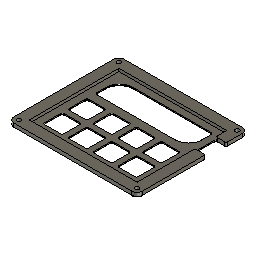
combined (Autodesk Fusion 360 archive; units mm, degrees)
design "Case_Lid"
Autodesk Fusion 360 part; units mm, degrees
sketch "plate-2025-12-06T19_36_10.325Z" plane through (0, 0, 0) normal (0, 0, 1) x (1, 0, 0)
  line L0 (3.275, -2.525) -> (15.775, -2.525)
  line L1 (3.275, -16.525) -> (15.775, -16.525)
  line L2 (2.525, -3.275) -> (2.525, -15.775)
  line L3 (16.525, -3.275) -> (16.525, -15.775)
  arc A0 (3.275, -2.525) -> (2.525, -3.275) centre (3.275, -3.275) ccw
  arc A1 (16.525, -3.275) -> (15.775, -2.525) centre (15.775, -3.275) ccw
  arc A2 (2.525, -15.775) -> (3.275, -16.525) centre (3.275, -15.775) ccw
  arc A3 (15.775, -16.525) -> (16.525, -15.775) centre (15.775, -15.775) ccw
  line L4 (22.325, -2.525) -> (34.825, -2.525)
  line L5 (22.325, -16.525) -> (34.825, -16.525)
  line L6 (21.575, -3.275) -> (21.575, -15.775)
  line L7 (35.575, -3.275) -> (35.575, -15.775)
  arc A4 (22.325, -2.525) -> (21.575, -3.275) centre (22.325, -3.275) ccw
  arc A5 (35.575, -3.275) -> (34.825, -2.525) centre (34.825, -3.275) ccw
  arc A6 (21.575, -15.775) -> (22.325, -16.525) centre (22.325, -15.775) ccw
  arc A7 (34.825, -16.525) -> (35.575, -15.775) centre (34.825, -15.775) ccw
  line L8 (41.375, -2.525) -> (53.875, -2.525)
  line L9 (41.375, -16.525) -> (53.875, -16.525)
  line L10 (40.625, -3.275) -> (40.625, -15.775)
  line L11 (54.625, -3.275) -> (54.625, -15.775)
  arc A8 (41.375, -2.525) -> (40.625, -3.275) centre (41.375, -3.275) ccw
  arc A9 (54.625, -3.275) -> (53.875, -2.525) centre (53.875, -3.275) ccw
  arc A10 (40.625, -15.775) -> (41.375, -16.525) centre (41.375, -15.775) ccw
  arc A11 (53.875, -16.525) -> (54.625, -15.775) centre (53.875, -15.775) ccw
  line L12 (60.425, -2.525) -> (72.925, -2.525)
  line L13 (60.425, -16.525) -> (72.925, -16.525)
  line L14 (59.675, -3.275) -> (59.675, -15.775)
  line L15 (73.675, -3.275) -> (73.675, -15.775)
  arc A12 (60.425, -2.525) -> (59.675, -3.275) centre (60.425, -3.275) ccw
  arc A13 (73.675, -3.275) -> (72.925, -2.525) centre (72.925, -3.275) ccw
  arc A14 (59.675, -15.775) -> (60.425, -16.525) centre (60.425, -15.775) ccw
  arc A15 (72.925, -16.525) -> (73.675, -15.775) centre (72.925, -15.775) ccw
  line L16 (3.275, -21.575) -> (15.775, -21.575)
  line L17 (3.275, -35.575) -> (15.775, -35.575)
  line L18 (2.525, -22.325) -> (2.525, -34.825)
  line L19 (16.525, -22.325) -> (16.525, -34.825)
  arc A16 (3.275, -21.575) -> (2.525, -22.325) centre (3.275, -22.325) ccw
  arc A17 (16.525, -22.325) -> (15.775, -21.575) centre (15.775, -22.325) ccw
  arc A18 (2.525, -34.825) -> (3.275, -35.575) centre (3.275, -34.825) ccw
  arc A19 (15.775, -35.575) -> (16.525, -34.825) centre (15.775, -34.825) ccw
  line L20 (22.325, -21.575) -> (34.825, -21.575)
  line L21 (22.325, -35.575) -> (34.825, -35.575)
  line L22 (21.575, -22.325) -> (21.575, -34.825)
  line L23 (35.575, -22.325) -> (35.575, -34.825)
  arc A20 (22.325, -21.575) -> (21.575, -22.325) centre (22.325, -22.325) ccw
  arc A21 (35.575, -22.325) -> (34.825, -21.575) centre (34.825, -22.325) ccw
  arc A22 (21.575, -34.825) -> (22.325, -35.575) centre (22.325, -34.825) ccw
  arc A23 (34.825, -35.575) -> (35.575, -34.825) centre (34.825, -34.825) ccw
  line L24 (41.375, -21.575) -> (53.875, -21.575)
  line L25 (41.375, -35.575) -> (53.875, -35.575)
  line L26 (40.625, -22.325) -> (40.625, -34.825)
  line L27 (54.625, -22.325) -> (54.625, -34.825)
  arc A24 (41.375, -21.575) -> (40.625, -22.325) centre (41.375, -22.325) ccw
  arc A25 (54.625, -22.325) -> (53.875, -21.575) centre (53.875, -22.325) ccw
  arc A26 (40.625, -34.825) -> (41.375, -35.575) centre (41.375, -34.825) ccw
  arc A27 (53.875, -35.575) -> (54.625, -34.825) centre (53.875, -34.825) ccw
  line L28 (60.425, -21.575) -> (72.925, -21.575)
  line L29 (60.425, -35.575) -> (72.925, -35.575)
  line L30 (59.675, -22.325) -> (59.675, -34.825)
  line L31 (73.675, -22.325) -> (73.675, -34.825)
  arc A28 (60.425, -21.575) -> (59.675, -22.325) centre (60.425, -22.325) ccw
  arc A29 (73.675, -22.325) -> (72.925, -21.575) centre (72.925, -22.325) ccw
  arc A30 (59.675, -34.825) -> (60.425, -35.575) centre (60.425, -34.825) ccw
  arc A31 (72.925, -35.575) -> (73.675, -34.825) centre (72.925, -34.825) ccw
  line L32 (-11.361, 35.925) -> (87.639, 35.925)
  line L33 (87.639, 35.925) -> (87.639, -49.075)
  line L34 (87.639, -49.075) -> (-11.361, -49.075)
  line L35 (-11.361, -49.075) -> (-11.361, 35.925)
  circle A32 centre (-7.361, 31.925) radius 1.6
  circle A33 centre (83.639, 31.925) radius 1.6
  circle A34 centre (83.639, -45.075) radius 1.6
  circle A35 centre (-7.361, -45.075) radius 1.6
  line L36 (73.753, 22.425) -> (12.525, 22.425)
  line L37 (2.525, 12.425) -> (2.525, 4.425)
  line L38 (2.525, 4.425) -> (63.753, 4.425)
  line L39 (73.753, 14.425) -> (73.753, 22.425)
  arc A36 (12.525, 22.425) -> (2.525, 12.425) centre (12.525, 12.425) ccw
  arc A37 (63.753, 4.425) -> (73.753, 14.425) centre (63.753, 14.425) ccw
  line L40 (-3.361, 27.925) -> (79.639, 27.925)
  line L41 (79.639, 27.925) -> (79.639, -41.075)
  line L42 (79.639, -41.075) -> (-3.361, -41.075)
  line L43 (-3.361, -41.075) -> (-3.361, 27.925)
  dimension "d1" = 99
  dimension "d2" = 85
  dimension "d3" = 13.886
  dimension "d4" = 13.5
  dimension "d12" = 3.2
  dimension "d13" = 4
  dimension "d14" = 4
  dimension "d15" = 3.2
  dimension "d16" = 4
  dimension "d17" = 4
  dimension "d18" = 3.2
  dimension "d19" = 3.2
  dimension "d20" = 4
  dimension "d21" = 4
  dimension "d22" = 4
  dimension "d23" = 4
  dimension "d34" = 13.886
  dimension "d36" = 13.886
  dimension "d37" = 18
  dimension "d38" = 13.5
  dimension "d39" = 10
  dimension "d40" = 10
  dimension "d47" = 8
  dimension "d48" = 8
  dimension "d49" = 8
  dimension "d50" = 8
  constraint horizontal L32
  constraint vertical L33
  constraint horizontal L34
  constraint vertical L35
  constraint horizontal L36
  constraint vertical L37
  constraint horizontal L38
  constraint vertical L39
  constraint tangent L36 A36
  constraint tangent L37 A36
  constraint tangent L38 A37
  constraint tangent L39 A37
  constraint horizontal L40
  constraint vertical L41
  constraint horizontal L42
  constraint vertical L43
  measures "d1" distance of L32.start L32.end
  measures "d2" distance of L32.start L34.end
  measures "d3" distance of L18 L35
  measures "d4" distance of L17 L34
  measures "d12" diameter of A32
  measures "d13" distance of L32 A32.centre
  measures "d14" distance of L35 A32.centre
  measures "d15" diameter of A33
  measures "d16" distance of L33 A33.centre
  measures "d17" distance of L32 A33.centre
  measures "d18" diameter of A35
  measures "d19" diameter of A34
  measures "d20" distance of L34 A34.centre
  measures "d21" distance of L33 A34.centre
  measures "d22" distance of L34 A35.centre
  measures "d23" distance of L35 A35.centre
  measures "d34" distance of L35 L37
  measures "d36" distance of L33 L39
  measures "d37" distance of L36 L38
  measures "d38" distance of L32 L36
  measures "d39" radius of A36
  measures "d40" radius of A37
  measures "d47" distance of L32 L40
  measures "d48" distance of L35 L43
  measures "d49" distance of L33 L41
  measures "d50" distance of L34 L42
extrude "Extrude1" add sketch "plate-2025-12-06T19_36_10.325Z" along normal blind 1.5 contours L32 L33 L34 L35 | L40 L41 L42 L43
extrude "Extrude2" add sketch "plate-2025-12-06T19_36_10.325Z" along normal blind 3.75 contours L32 L33 L34 L35
sketch "Sketch2" plane through (0, 0, 3.75) normal (0, 0, 1) x (-1, 0, 0)
  circle A0 centre (-83.639, -31.925) radius 1.6
  circle A1 centre (7.361, 45.075) radius 1.6
  line L0 (-79.639, 41.075) -> (3.361, 41.075)
  line L1 (3.361, 41.075) -> (3.361, -27.925)
  line L2 (3.361, -27.925) -> (-79.639, -27.925)
  line L3 (-79.639, -27.925) -> (-79.639, 41.075)
  circle A2 centre (-83.639, 45.075) radius 1.6
  circle A3 centre (7.361, -31.925) radius 1.6
  line L4 (11.361, 49.075) -> (-87.639, 49.075)
  line L5 (-87.639, 49.075) -> (-87.639, -35.925)
  line L6 (-87.639, -35.925) -> (11.361, -35.925)
  line L7 (11.361, -35.925) -> (11.361, 49.075)
  line L8 (-79.639, -19.549) -> (-87.639, -19.549)
  line L9 (-87.639, -19.549) -> (-87.639, -3.549)
  line L10 (-87.639, -3.549) -> (-79.639, -3.549)
  line L11 (-79.639, -3.549) -> (-79.639, -19.549)
  dimension "d67" = 16.376
  dimension "d68" = 52.624
  constraint horizontal L8
  constraint vertical L9
  constraint horizontal L10
  constraint vertical L11
  constraint coincident L5 L9.end
  constraint coincident L3 L8.start
  measures "d67" distance of L6 L8
  measures "d68" distance of L4 L10
extrude "Extrude4" cut sketch "Sketch2" against normal blind 5 contours L3 L5 L8 L9 L10 L11
fillet "Fillet11" radius 1 4 edges at (73.753, 22.425, 0.75) (2.525, 4.425, 0.75) (79.639, 3.549, 0.75) (79.639, 19.549, 0.75)
fillet "Fillet8" radius 4 4 edges at (87.639, 35.925, 1.875) (87.639, -49.075, 1.875) (-11.361, 35.925, 1.875) (-11.361, -49.075, 1.875)
fillet "Fillet9" radius 1 90 edges at (2.525, 8.925, 0) (5.4539, 19.4961, 0) (42.639, 22.425, 0) (73.4601, 22.1321, 0) (73.753, 17.925, 0) (70.8241, 7.3539, 0) (33.639, 4.425, 0) (2.8179, 4.7179, 0) (16.525, -9.525, 0) (16.3053, -16.3053, 0) (9.525, -16.525, 0) (2.7447, -16.3053, 0) (2.525, -9.525, 0) (2.7447, -2.7447, 0) (9.525, -2.525, 0) (16.3053, -2.7447, 0) (35.575, -9.525, 0) (35.3553, -16.3053, 0) (28.575, -16.525, 0) (21.7947, -16.3053, 0) (21.575, -9.525, 0) (21.7947, -2.7447, 0) (28.575, -2.525, 0) (35.3553, -2.7447, 0) (54.625, -9.525, 0) (54.4053, -16.3053, 0) (47.625, -16.525, 0) (40.8447, -16.3053, 0) (40.625, -9.525, 0) (40.8447, -2.7447, 0) (47.625, -2.525, 0) (54.4053, -2.7447, 0) (73.675, -9.525, 0) (73.4553, -16.3053, 0) (66.675, -16.525, 0) (59.8947, -16.3053, 0) (59.675, -9.525, 0) (59.8947, -2.7447, 0) (66.675, -2.525, 0) (73.4553, -2.7447, 0) (59.675, -28.575, 0) (59.8947, -21.7947, 0) (66.675, -21.575, 0) (73.4553, -21.7947, 0) (73.675, -28.575, 0) (73.4553, -35.3553, 0) (66.675, -35.575, 0) (59.8947, -35.3553, 0) (40.625, -28.575, 0) (40.8447, -21.7947, 0) (47.625, -21.575, 0) (54.4053, -21.7947, 0) (54.625, -28.575, 0) (54.4053, -35.3553, 0) (47.625, -35.575, 0) (40.8447, -35.3553, 0) (21.575, -28.575, 0) (21.7947, -21.7947, 0) (28.575, -21.575, 0) (35.3553, -21.7947, 0) (35.575, -28.575, 0) (35.3553, -35.3553, 0) (28.575, -35.575, 0) (21.7947, -35.3553, 0) (2.525, -28.575, 0) (2.7447, -21.7947, 0) (9.525, -21.575, 0) (16.3053, -21.7947, 0) (16.525, -28.575, 0) (16.3053, -35.3553, 0) (9.525, -35.575, 0) (2.7447, -35.3553, 0) (86.4674, 34.7534, 0) (38.139, 35.925, 0) (-10.1894, 34.7534, 0) (-11.361, -6.575, 0) (-10.1894, -47.9034, 0) (38.139, -49.075, 0) (86.4674, -47.9034, 0) (87.639, -20.763, 0) (87.639, 25.737, 0) (84.139, 19.549, 0) (79.9319, 19.2561, 0) (79.639, 11.549, 0) (79.9319, 3.8419, 0) (84.139, 3.549, 0) (87.639, 3.549, 1.875) (87.639, 19.549, 1.875) (79.639, 3.549, 2.625) (79.639, 19.549, 2.625)
fillet "Fillet12" radius 0.4 75 edges at (59.675, -28.575, 1.5) (59.8947, -21.7947, 1.5) (66.675, -21.575, 1.5) (73.4553, -21.7947, 1.5) (73.675, -28.575, 1.5) (73.4553, -35.3553, 1.5) (66.675, -35.575, 1.5) (59.8947, -35.3553, 1.5) (40.625, -28.575, 1.5) (40.8447, -21.7947, 1.5) (47.625, -21.575, 1.5) (54.4053, -21.7947, 1.5) (54.625, -28.575, 1.5) (54.4053, -35.3553, 1.5) (47.625, -35.575, 1.5) (40.8447, -35.3553, 1.5) (21.575, -28.575, 1.5) (21.7947, -21.7947, 1.5) (28.575, -21.575, 1.5) (35.3553, -21.7947, 1.5) (35.575, -28.575, 1.5) (35.3553, -35.3553, 1.5) (28.575, -35.575, 1.5) (21.7947, -35.3553, 1.5) (2.525, -28.575, 1.5) (2.7447, -21.7947, 1.5) (9.525, -21.575, 1.5) (16.3053, -21.7947, 1.5) (16.525, -28.575, 1.5) (16.3053, -35.3553, 1.5) (9.525, -35.575, 1.5) (2.7447, -35.3553, 1.5) (2.525, -9.525, 1.5) (2.7447, -2.7447, 1.5) (9.525, -2.525, 1.5) (16.3053, -2.7447, 1.5) (16.525, -9.525, 1.5) (16.3053, -16.3053, 1.5) (9.525, -16.525, 1.5) (2.7447, -16.3053, 1.5) (21.575, -9.525, 1.5) (21.7947, -2.7447, 1.5) (28.575, -2.525, 1.5) (35.3553, -2.7447, 1.5) (35.575, -9.525, 1.5) (35.3553, -16.3053, 1.5) (28.575, -16.525, 1.5) (21.7947, -16.3053, 1.5) (40.625, -9.525, 1.5) (40.8447, -2.7447, 1.5) (47.625, -2.525, 1.5) (54.4053, -2.7447, 1.5) (54.625, -9.525, 1.5) (54.4053, -16.3053, 1.5) (47.625, -16.525, 1.5) (40.8447, -16.3053, 1.5) (59.675, -9.525, 1.5) (59.8947, -2.7447, 1.5) (66.675, -2.525, 1.5) (73.4553, -2.7447, 1.5) (73.675, -9.525, 1.5) (73.4553, -16.3053, 1.5) (66.675, -16.525, 1.5) (59.8947, -16.3053, 1.5) (2.8179, 4.7179, 1.5) (2.525, 8.925, 1.5) (5.4539, 19.4961, 1.5) (42.639, 22.425, 1.5) (73.4601, 22.1321, 1.5) (73.753, 17.925, 1.5) (70.8241, 7.3539, 1.5) (33.639, 4.425, 1.5) (79.9319, 3.8419, 1.5) (79.639, 11.549, 1.5) (79.9319, 19.2561, 1.5)
equation "d1 = 8 mm + 8 mm + 83 mm"
equation "d2 = 8 mm + 8 mm + 69 mm"
equation "d3 = 9.5 mm + 4.386 mm"
equation "d4 = 9.5 mm + 4 mm"
equation "d51 = 1.5 mm + 2.25 mm"

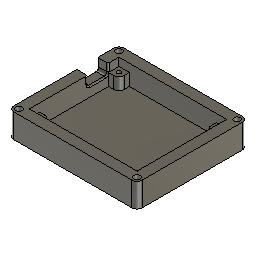
design "Case_Base"
Autodesk Fusion 360 part; units mm, degrees
sketch "Sketch1" plane through (0, 0, 0) normal (0, 0, 1) x (1, 0, 0) in component "Hackpad Case"
  line L0 (1, 47.0118) -> (84, 47.0118)
  line L1 (84, 47.0118) -> (84, -21.9882)
  line L2 (84, -21.9882) -> (1, -21.9882)
  line L3 (1, -21.9882) -> (1, 47.0118)
  line L4 (-7, 55.0118) -> (92, 55.0118)
  line L5 (92, 55.0118) -> (92, -29.9882)
  line L6 (92, -29.9882) -> (-7, -29.9882)
  line L7 (-7, -29.9882) -> (-7, 55.0118)
  circle A0 centre (-3, 51.0118) radius 2.35
  circle A1 centre (88, 51.0118) radius 2.35
  circle A2 centre (-3, -25.9882) radius 2.35
  circle A3 centre (88, -25.9882) radius 2.35
  circle A4 centre (4.9559, 43.136) radius 1.6
  line L8 (1, 47.0118) -> (9, 47.0118)
  line L9 (9, 47.0118) -> (9, 43.0118)
  line L10 (5, 39.0118) -> (1, 39.0118)
  line L11 (1, 39.0118) -> (1, 47.0118)
  circle A5 centre (79.9559, 43.136) radius 1.6
  line L12 (84, 47.0118) -> (76, 47.0118)
  line L13 (76, 47.0118) -> (76, 43.0118)
  line L14 (80, 39.0118) -> (84, 39.0118)
  line L15 (84, 39.0118) -> (84, 47.0118)
  circle A6 centre (4.9559, -17.864) radius 1.6
  line L16 (1, -21.9882) -> (9, -21.9882)
  line L17 (9, -21.9882) -> (9, -17.9882)
  line L18 (5, -13.9882) -> (1, -13.9882)
  line L19 (1, -13.9882) -> (1, -21.9882)
  line L20 (84, -21.9882) -> (76, -21.9882)
  line L21 (76, -21.9882) -> (76, -17.9882)
  line L22 (80, -13.9882) -> (84, -13.9882)
  line L23 (84, -13.9882) -> (84, -21.9882)
  circle A7 centre (79.9559, -17.864) radius 1.6
  arc A8 (5, 39.0118) -> (9, 43.0118) centre (5, 43.0118) ccw
  arc A9 (76, 43.0118) -> (80, 39.0118) centre (80, 43.0118) ccw
  arc A10 (80, -13.9882) -> (76, -17.9882) centre (80, -17.9882) ccw
  arc A11 (9, -17.9882) -> (5, -13.9882) centre (5, -17.9882) ccw
  point P0 (9, 39.0118)
  point P1 (76, 39.0118)
  point P2 (9, -13.9882)
  point P3 (76, -13.9882)
  dimension "d1" = 83
  dimension "d2" = 69
  dimension "d3" = 8
  dimension "d4" = 8
  dimension "d5" = 8
  dimension "d6" = 8
  dimension "d7" = 4.7
  dimension "d8" = 4
  dimension "d9" = 4
  dimension "d10" = 4.7
  dimension "d11" = 4
  dimension "d12" = 4
  dimension "d13" = 4.7
  dimension "d14" = 4
  dimension "d15" = 4
  dimension "d16" = 4.7
  dimension "d17" = 4
  dimension "d18" = 4
  dimension "d22" = 3.2
  dimension "d25" = 8
  dimension "d26" = 8
  dimension "d27" = 3.2
  dimension "d28" = 8
  dimension "d29" = 8
  dimension "d32" = 3.2
  dimension "d33" = 8
  dimension "d34" = 8
  dimension "d37" = 8
  dimension "d38" = 8
  dimension "d39" = 3.2
  dimension "d62" = 61
  dimension "d63" = 75
  dimension "d64" = 75
  dimension "d65" = 61
  dimension "d66" = 4
  dimension "d67" = 4
  dimension "d68" = 4
  dimension "d69" = 4
  constraint horizontal L0
  constraint vertical L1
  constraint horizontal L2
  constraint vertical L3
  constraint horizontal L4
  constraint vertical L5
  constraint horizontal L6
  constraint vertical L7
  constraint horizontal L8
  constraint vertical L9
  constraint horizontal L10
  constraint vertical L11
  constraint horizontal L12
  constraint vertical L13
  constraint horizontal L14
  constraint vertical L15
  constraint horizontal L16
  constraint vertical L17
  constraint horizontal L18
  constraint vertical L19
  constraint horizontal L20
  constraint vertical L21
  constraint horizontal L22
  constraint vertical L23
  constraint coincident P0 L9
  constraint coincident P0 L10
  constraint tangent L9 A8
  constraint tangent L10 A8
  constraint coincident P1 L13
  constraint coincident P1 L14
  constraint tangent L13 A9
  constraint tangent L14 A9
  constraint coincident P3 L21
  constraint coincident P3 L22
  constraint tangent L21 A10
  constraint tangent L22 A10
  constraint coincident P2 L18
  constraint coincident P2 L17
  constraint tangent L18 A11
  constraint tangent L17 A11
  measures "d1" distance of L0.start L0.end
  measures "d2" distance of L0.start L2.end
  measures "d3" distance of L0 L4
  measures "d4" distance of L2 L6
  measures "d5" distance of L1 L5
  measures "d6" distance of L3 L7
  measures "d7" diameter of A0
  measures "d8" distance of L7 A0.centre
  measures "d9" distance of L4 A0.centre
  measures "d10" diameter of A1
  measures "d11" distance of L4 A1.centre
  measures "d12" distance of L5 A1.centre
  measures "d13" diameter of A2
  measures "d14" distance of L7 A2.centre
  measures "d15" distance of L6 A2.centre
  measures "d16" diameter of A3
  measures "d17" distance of L5 A3.centre
  measures "d18" distance of L6 A3.centre
  measures "d22" diameter of A4
  measures "d25" distance of L8.end P0
  measures "d26" distance of P0 L10.end
  measures "d27" diameter of A5
  measures "d28" distance of P1 L14.end
  measures "d29" distance of L12.end P1
  measures "d32" diameter of A6
  measures "d33" distance of P2 L18.end
  measures "d34" distance of L16.end P2
  measures "d37" distance of P3 L22.end
  measures "d38" distance of L20.end P3
  measures "d39" diameter of A7
  measures "d62" distance of A4.centre A6.centre
  measures "d63" distance of A4.centre A5.centre
  measures "d64" distance of A6.centre A7.centre
  measures "d65" distance of A5.centre A7.centre
  measures "d66" radius of A8
  measures "d67" radius of A9
  measures "d68" radius of A10
  measures "d69" radius of A11
extrude "Extrude1" add sketch "Sketch1" along normal blind 3 contours L0 L3 L8 L9 L10 L11 A8 | L0 L1 L2 L3 L9 L10 L13 L14 L17 L18 L21 L22 A8 A9 A10 A11 | L0 L1 L12 L13 L14 L15 A9 | L2 L3 L16 L17 L18 L19 A11 | L1 L2 L20 L21 L22 L23 A10 | L4 L5 L6 L7 | A0 | A1 | A2 | A3
extrude "Extrude2" add sketch "Sketch1" along normal blind 18.5 contours L4 L5 L6 L7
extrude "Extrude3" add sketch "Sketch1" along normal blind 12.31 contours L0 L3 L8 L9 L10 L11 A8 | L0 L1 L12 L13 L14 L15 A9 | L2 L3 L16 L17 L18 L19 A11 | L1 L2 L20 L21 L22 L23 A10
sketch "Sketch3" plane through (0, 0, 18.5) normal (0, 0, 1) x (-1, 0, 0)
  line L0 (-84, -47.0118) -> (-84, 21.9882)
  line L1 (-84, 21.9882) -> (-1, 21.9882)
  line L2 (-1, 21.9882) -> (-1, -47.0118)
  line L3 (-1, -47.0118) -> (-84, -47.0118)
  circle A0 centre (3, 25.9882) radius 2.35
  circle A1 centre (-88, 25.9882) radius 2.35
  circle A2 centre (-88, -51.0118) radius 2.35
  circle A3 centre (3, -51.0118) radius 2.35
  line L4 (7, 29.9882) -> (-92, 29.9882)
  line L5 (-92, 29.9882) -> (-92, -55.0118)
  line L6 (-92, -55.0118) -> (7, -55.0118)
  line L7 (7, -55.0118) -> (7, 29.9882)
  line L8 (7, -38.636) -> (-1, -38.636)
  line L9 (-1, -38.636) -> (-1, -22.636)
  line L10 (-1, -22.636) -> (7, -22.636)
  line L11 (7, -22.636) -> (7, -38.636)
  circle A4 centre (-4.9559, -43.136) radius 1.6
  circle A5 centre (-4.9559, 17.864) radius 1.6
  dimension "d78" = 4.5
  dimension "d79" = 40.5
  constraint horizontal L8
  constraint vertical L9
  constraint horizontal L10
  constraint vertical L11
  constraint coincident L2 L9.end
  constraint coincident L7 L8.start
  measures "d78" distance of L8 A4.centre
  measures "d79" distance of L10 A5.centre
extrude "Extrude4" cut sketch "Sketch3" against normal blind 8 contours L2 L7 L8 L9 L10 L11
fillet "Fillet2" radius 4 4 edges at (-7, -29.9882, 9.25) (92, -29.9882, 9.25) (92, 55.0118, 9.25) (-7, 55.0118, 9.25)
fillet "Fillet3" radius 2 2 edges at (-3, 22.636, 10.5) (-3, 38.636, 10.5)
fillet "Fillet4" radius 1 10 edges at (-7, 22.636, 15.5) (-7, 23.2217, 11.0858) (-7, 30.636, 10.5) (-7, 38.0502, 11.0858) (-7, 38.636, 15.5) (1, 38.636, 15.5) (1, 38.0502, 11.0858) (1, 30.636, 10.5) (1, 23.2217, 11.0858) (1, 22.636, 15.5)
component "Hackpad Case" placed x (1, 0, 0) y (0, 1, 0) z (0, 0, 1) at (0, 0, 0)
